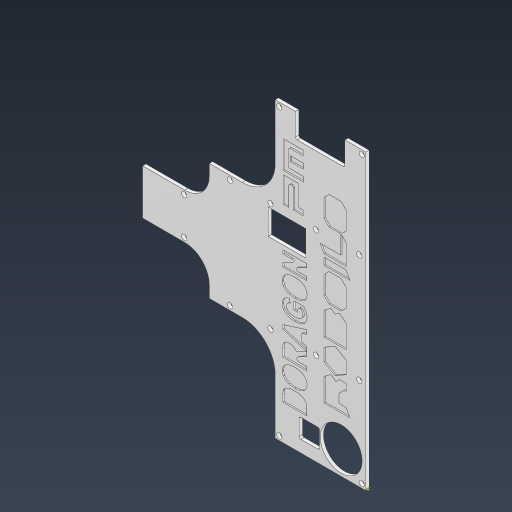
# Autodesk Inventor part: ceil
Saved by Autodesk Inventor 2023 (Build 270158000, 158)
## iProperties
Created: 2024-05-26
Part Number: ceil
Material: ABS Plastic
Document SubType Name: Modeling
Designer: szymo
Density: 1.06 g/cm^3
Appearance: Smooth - White
Mass: 26.6149 g
Surface Area: 293.171 cm^2
Volume: 25.1084 cm^3
TOTAL MASS: 0.0
Author: szymo
Autodesk Inventor part; units mm, degrees
ref_plane "YZ Plane" through (0, 0, 0) normal (1, 0, 0) x (0, 1, 0)
ref_plane "XZ Plane" through (0, 0, 0) normal (0, 1, 0) x (-1, 0, 0)
ref_plane "Work Plane1" through (-50.5, 0, 0) normal (0, 0, 1) x (1, 0, 0)
sketch "Sketch3" plane through (-50.5, 0, 0) normal (0, 0, 1) x (1, 0, 0)
  line L0 (135.5648, 0) -> (135.5648, 5.2284) projected
  line L1 (0, 5) -> (134.493, 5) projected
  line L2 (0, 0) -> (0, 5) projected
  line L3 (0, 71) -> (135.5648, 71) projected
  line L4 (0, 71) -> (0, 66) projected
  line L5 (0, 66) -> (135.5648, 66) projected
  line L6 (135.5648, 71) -> (135.5648, 66) projected
  line L7 (131.5648, 119.5) -> (134.5648, 119.5) projected
  line L8 (135.5648, 124.5) -> (135.5648, 120.5) projected
  line L9 (135.5648, 124.5) -> (51.5, 124.5) projected
  line L10 (86.5, 123.5) -> (129.5648, 123.5) projected
  line L11 (80.5, 122.5) -> (80.5, 120.5) projected
  line L12 (81.5, 119.5) -> (84.5, 119.5) projected
  line L13 (85.5, 122.5) -> (85.5, 120.5) projected
  line L14 (51.5, 123.5) -> (79.5, 123.5) projected
  line L15 (130.5648, 122.5) -> (130.5648, 120.5) projected
  line L16 (120.8148, 112) -> (120.8148, 123) projected
  line L17 (120.8148, 123) -> (94.8148, 123) projected
  line L18 (94.8148, 123) -> (94.8148, 112) projected
  line L19 (94.8148, 112) -> (120.8148, 112) projected
  line L20 (130.5648, -51.5) -> (130.5648, -49.5) projected
  line L21 (51.5, -52.5) -> (79.5, -52.5) projected
  line L22 (85.5, -51.5) -> (85.5, -49.5) projected
  line L23 (131.5648, -48.5) -> (134.5648, -48.5) projected
  line L24 (80.5, -51.5) -> (80.5, -49.5) projected
  line L25 (86.5, -52.5) -> (129.5648, -52.5) projected
  line L26 (135.5648, -53.5) -> (51.5, -53.5) projected
  line L27 (135.5648, -53.5) -> (135.5648, -49.5) projected
  line L28 (81.5, -48.5) -> (84.5, -48.5) projected
  line L29 (95.5648, -45.8) -> (95.5648, -35.2) projected
  line L30 (106.8648, -35.2) -> (95.5648, -35.2) projected
  line L31 (106.8648, -35.2) -> (106.8648, -45.8) projected
  line L32 (95.5648, -45.8) -> (106.8648, -45.8) projected
  circle A0 centre (90.4898, -49.075) radius 1.675 projected
  circle A1 centre (124.5398, -49.075) radius 1.675 projected
  line L33 (126.3648, -33.5) -> (126.3648, -45.5) projected
  line L34 (126.3648, -45.5) -> (114.7648, -45.5) projected
  line L35 (114.7648, -45.5) -> (114.7648, -33.5) projected
  line L36 (114.7648, -33.5) -> (86.8648, -33.5) projected
  line L37 (86.8648, -33.5) -> (86.8648, -52.5) projected
  line L38 (86.8648, -52.5) -> (128.0648, -52.5) projected
  line L39 (128.0648, -52.5) -> (128.0648, -33.5) projected
  line L40 (128.0648, -33.5) -> (126.3648, -33.5) projected
  line L41 (126.3648, -32.7) -> (114.7648, -32.7) projected
  line L42 (114.7648, -32.7) -> (114.7648, -45.5) projected
  line L43 (114.7648, -45.5) -> (126.3648, -45.5) projected
  line L44 (126.3648, -45.5) -> (126.3648, -32.7) projected
  line L45 (80.5, -53.5) -> (135.5648, -53.5)
  line L46 (135.5648, -53.5) -> (135.5648, 124.5)
  line L47 (135.5648, 124.5) -> (80.5, 124.5)
  line L48 (80.5, 124.5) -> (80.5, -53.5)
  line L49 (0, 22) -> (80.5, 22)
  line L50 (80.5, 22) -> (80.5, 49.5)
  line L51 (80.5, 49.5) -> (0, 49.5)
  line L52 (0, 49.5) -> (0, 22)
  line L53 (80.5, 22) -> (50.5, 22)
  line L54 (50.5, 22) -> (50.5, 0)
  line L55 (50.5, 0) -> (80.5, 0)
  line L56 (80.5, 0) -> (80.5, 22)
  line L57 (80.5, 46.5815) -> (80.5, 71)
  line L58 (80.5, 71) -> (50.5, 71)
  line L59 (50.5, 71) -> (50.5, 49.5)
  arc A2 (97.9124, 50.9) -> (98.0124, 51) centre (97.9124, 51) ccw projected
  line L60 (77.4124, 50.9) -> (97.9124, 50.9) projected
  arc A3 (77.3124, 51) -> (77.4124, 50.9) centre (77.4124, 51) ccw projected
  line L61 (77.3124, 65.5) -> (77.3124, 51) projected
  arc A4 (77.4124, 65.6) -> (77.3124, 65.5) centre (77.4124, 65.5) ccw projected
  line L62 (97.9124, 65.6) -> (77.4124, 65.6) projected
  arc A5 (98.0124, 65.5) -> (97.9124, 65.6) centre (97.9124, 65.5) ccw projected
  line L63 (98.0124, 51) -> (98.0124, 65.5) projected
  line L64 (96.2124, 63.7) -> (96.2124, 52.8) projected
  arc A6 (96.2124, 63.7) -> (95.9124, 64) centre (95.9124, 63.7) ccw projected
  line L65 (95.9124, 64) -> (95.8124, 64) projected
  line L66 (95.8124, 64) -> (95.3509, 64.55) projected
  line L67 (95.3509, 64.55) -> (94.9739, 64.55) projected
  line L68 (94.9739, 64.55) -> (94.5124, 64) projected
  line L69 (94.5124, 64) -> (90.8124, 64) projected
  line L70 (90.8124, 64) -> (90.8124, 64.35) projected
  line L71 (90.8124, 64.35) -> (89.5124, 64.35) projected
  line L72 (89.5124, 64) -> (89.5124, 64.35) projected
  line L73 (89.5124, 64) -> (85.8124, 64) projected
  line L74 (85.8124, 64) -> (85.8124, 64.35) projected
  line L75 (85.8124, 64.35) -> (84.5124, 64.35) projected
  line L76 (84.5124, 64) -> (84.5124, 64.35) projected
  line L77 (84.5124, 64) -> (80.8124, 64) projected
  line L78 (80.8124, 64) -> (80.3509, 64.55) projected
  line L79 (80.3509, 64.55) -> (79.9739, 64.55) projected
  line L80 (79.9739, 64.55) -> (79.5124, 64) projected
  line L81 (79.5124, 64) -> (79.4124, 64) projected
  arc A7 (79.4124, 64) -> (79.1124, 63.7) centre (79.4124, 63.7) ccw projected
  line L82 (79.1124, 63.7) -> (79.1124, 52.8) projected
  arc A8 (79.1124, 52.8) -> (79.4124, 52.5) centre (79.4124, 52.8) ccw projected
  line L83 (79.4124, 52.5) -> (79.5124, 52.5) projected
  line L84 (79.5124, 52.5) -> (79.9739, 51.95) projected
  line L85 (80.3509, 51.95) -> (79.9739, 51.95) projected
  line L86 (80.3509, 51.95) -> (80.8124, 52.5) projected
  line L87 (80.8124, 52.5) -> (84.5124, 52.5) projected
  line L88 (84.5124, 52.5) -> (84.5124, 52.15) projected
  line L89 (85.8124, 52.15) -> (84.5124, 52.15) projected
  line L90 (85.8124, 52.5) -> (85.8124, 52.15) projected
  line L91 (85.8124, 52.5) -> (89.5124, 52.5) projected
  line L92 (89.5124, 52.5) -> (89.5124, 52.15) projected
  line L93 (90.8124, 52.15) -> (89.5124, 52.15) projected
  line L94 (90.8124, 52.5) -> (90.8124, 52.15) projected
  line L95 (90.8124, 52.5) -> (94.5124, 52.5) projected
  line L96 (94.5124, 52.5) -> (94.9739, 51.95) projected
  line L97 (95.3509, 51.95) -> (94.9739, 51.95) projected
  line L98 (95.3509, 51.95) -> (95.8124, 52.5) projected
  line L99 (95.8124, 52.5) -> (95.9124, 52.5) projected
  arc A9 (95.9124, 52.5) -> (96.2124, 52.8) centre (95.9124, 52.8) ccw projected
  line L100 (78.1624, 55.35) -> (78.8624, 55.35) projected
  line L101 (78.8624, 55.35) -> (78.8624, 61.15) projected
  line L102 (78.1624, 61.15) -> (78.8624, 61.15) projected
  line L103 (78.1624, 61.15) -> (78.1624, 55.35) projected
  line L104 (97.1624, 61.15) -> (97.1624, 55.35) projected
  line L105 (96.4624, 61.15) -> (97.1624, 61.15) projected
  line L106 (96.4624, 55.35) -> (96.4624, 61.15) projected
  line L107 (96.4624, 55.35) -> (97.1624, 55.35) projected
  arc A10 (76.8124, 51) -> (77.4124, 50.4) centre (77.4124, 51) ccw
  line L108 (77.4124, 50.4) -> (97.9124, 50.4)
  arc A11 (97.9124, 50.4) -> (98.5124, 51) centre (97.9124, 51) ccw
  line L109 (98.5124, 51) -> (98.5124, 65.5)
  arc A12 (98.5124, 65.5) -> (97.9124, 66.1) centre (97.9124, 65.5) ccw
  line L110 (97.9124, 66.1) -> (77.4124, 66.1)
  arc A13 (77.4124, 66.1) -> (76.8124, 65.5) centre (77.4124, 65.5) ccw
  line L111 (76.8124, 65.5) -> (76.8124, 51)
  line L112 (95.0648, -34.7) -> (95.0648, -46.3)
  line L113 (95.0648, -46.3) -> (107.3648, -46.3)
  line L114 (107.3648, -46.3) -> (107.3648, -34.7)
  line L115 (107.3648, -34.7) -> (95.0648, -34.7)
  line L116 (114.2648, -45.5) -> (114.2648, -32.2)
  line L117 (114.2648, -32.2) -> (126.8648, -32.2)
  line L118 (126.8648, -32.2) -> (126.8648, -45.5)
  line L119 (126.3648, -46) -> (114.7648, -46)
  line L120 (92.8148, 110) -> (92.8148, 125)
  line L121 (92.8148, 125) -> (122.8148, 125)
  line L122 (122.8148, 125) -> (122.8148, 110)
  line L123 (122.8148, 110) -> (92.8148, 110)
  line L124 (114.2648, -45.5) -> (114.2648, -46)
  line L125 (114.2648, -46) -> (114.7648, -46)
  line L126 (126.3648, -46) -> (126.8648, -46)
  line L127 (126.8648, -46) -> (126.8648, -45.5)
  line L128 (51.5, -53.5) -> (51.5, -52.5) projected
  line L129 (51.5, 124.5) -> (51.5, 123.5) projected
  circle A14 centre (105.3205, 68.5) radius 1.75 projected
  circle A15 centre (53, 68.5) radius 1.75 projected
  circle A16 centre (77.648, 2.5) radius 1.75 projected
  circle A17 centre (131.5519, 2.5) radius 1.75 projected
  line L130 (50.5, 27) -> (0, 27) projected
  line L131 (0, 27) -> (0, 22) projected
  line L132 (50.5, 22) -> (0, 22) projected
  line L133 (50.5, 27) -> (50.5, 22) projected
  line L134 (50.5, 44.5) -> (0, 44.5) projected
  line L135 (50.5, 44.5) -> (50.5, 49.5) projected
  line L136 (50.5, 49.5) -> (0, 49.5) projected
  line L137 (0, 44.5) -> (0, 49.5) projected
  line L138 (50.5, 0) -> (40.5, 0)
  line L139 (40.5, 0) -> (40.5, 22)
  line L140 (40.5, 22) -> (50.5, 22)
  line L141 (50.5, 22) -> (50.5, 0)
  line L142 (50.5, 49.5) -> (40.5, 49.5)
  line L143 (40.5, 49.5) -> (40.5, 71)
  line L144 (40.5, 71) -> (50.5, 71)
  line L145 (50.5, 71) -> (50.5, 49.5)
  ellipse E0 centre (134.493, 7) end of major axis (136.8024, 7) minor radius 2 (134.493, 5) -> (135.5648, 5.2284) ccw projected
  circle A18 centre (25.25, 47) radius 1.75 projected
  circle A19 centre (25.25, 24.5) radius 1.75 projected
  line L146 (0, 0) -> (3.5, 0) projected
  line L147 (3.5, 0) -> (47, 0) projected
  line L148 (47, 0) -> (135.5648, 0) projected
  circle A20 centre (105.3205, 2.5) radius 1.75 projected
  circle A21 centre (53, 2.5) radius 1.75 projected
  arc A22 (81.5, -48.5) -> (80.5, -49.5) centre (81.5, -49.5) ccw projected
  arc A23 (79.5, -52.5) -> (80.5, -51.5) centre (79.5, -51.5) ccw projected
  arc A24 (135.5648, -49.5) -> (134.5648, -48.5) centre (134.5648, -49.5) ccw projected
  arc A25 (131.5648, -48.5) -> (130.5648, -49.5) centre (131.5648, -49.5) ccw projected
  arc A26 (129.5648, -52.5) -> (130.5648, -51.5) centre (129.5648, -51.5) ccw projected
  arc A27 (85.5, -51.5) -> (86.5, -52.5) centre (86.5, -51.5) ccw projected
  arc A28 (85.5, -49.5) -> (84.5, -48.5) centre (84.5, -49.5) ccw projected
  circle A29 centre (133.0648, -51) radius 1.75 projected
  circle A30 centre (83, -51) radius 1.75 projected
  arc A31 (86.5, 123.5) -> (85.5, 122.5) centre (86.5, 122.5) ccw projected
  arc A32 (130.5648, 122.5) -> (129.5648, 123.5) centre (129.5648, 122.5) ccw projected
  arc A33 (134.5648, 119.5) -> (135.5648, 120.5) centre (134.5648, 120.5) ccw projected
  arc A34 (80.5, 120.5) -> (81.5, 119.5) centre (81.5, 120.5) ccw projected
  arc A35 (84.5, 119.5) -> (85.5, 120.5) centre (84.5, 120.5) ccw projected
  arc A36 (130.5648, 120.5) -> (131.5648, 119.5) centre (131.5648, 120.5) ccw projected
  arc A37 (80.5, 122.5) -> (79.5, 123.5) centre (79.5, 122.5) ccw projected
  circle A38 centre (133.0648, 122) radius 1.75 projected
  circle A39 centre (83, 122) radius 1.75 projected
  point P0 (122.8148, 124.5)
  point P1 (92.8148, 124.5)
  point P2 (0, 44)
  point P3 (50.5, 44)
  point P4 (122.8148, 124.5)
  point P5 (122.8148, 123.5)
  point P6 (92.8148, 123.5)
  point P7 (92.8148, 124.5)
  point P8 (80.5, 123.5)
  point P9 (50.5, 66)
  point P10 (50.5, 5)
  point P11 (80.5, -52.5)
  point P12 (80.5, 66)
  point P13 (80.5, 5)
  point P14 (135.5648, 5)
  point P15 (80.5, 22)
  point P16 (50.5, 27)
  point P17 (0, 27)
  point P18 (80.5, -51.5)
  point P19 (77.0807, 66)
  point P20 (80.5, 66.1)
  point P21 (135.5648, 5.2284)
  point P22 (80.5, 50.4)
  point P23 (40.5, 5)
  point P24 (135.5648, 119.5)
  point P25 (80.5, 119.5)
  dimension "d16" = 0.5
  dimension "d17" = 0.5
  dimension "d18" = 0.5
  dimension "d19" = 0.5
  dimension "d20" = 2
  dimension "d191" = 10
  dimension "d192" = 10
  constraints: 86 end point, 12 parallel, 8 point on circle, 7 perpendicular, 7 point on line, 6 horizontal, 4 centre point, 2 collinear, 2 vertical, 17 other
  measures "d16" distance between parallel lines of L61 L111
  measures "d17" distance between parallel lines of L29 L112
  measures "d18" distance between parallel lines of L42 L116
  measures "d19" distance between parallel lines of L34 L119
  measures "d20" distance between parallel lines of L18 L120
  measures "d191" distance between parallel lines of L139 L54
  measures "d192" distance between parallel lines of L59 L143
extrude "Extrusion2" add sketch "Sketch3" along normal blind 2 contours L148 L48 L1 E0 L0 | L46 A24 L23 A25 L20 A26 L25 L39 L40 L118 L117 L116 L36 L37 A27 L22 A28 L28 A22 L48 L148 | E0 L1 L48 L108 A11 L109 A12 L5 L46 | L27 L26 L48 L24 A22 L28 A28 L22 A27 L25 A26 L20 A25 L23 A24 | L55 L54 L1 L48 | L5 A12 L110 L48 L3 L6 | L1 L54 L49 L48 | L138 L139 L1 L54 | A12 L109 A11 L108 L48 L60 A2 L63 A5 L62 L5 | L5 L48 L110 A12 | L3 L48 A34 L12 A35 L13 A31 L10 L120 L123 L122 A32 L15 A36 L7 A33 L46 | L1 L139 L49 L54 | L49 L133 L130 L52 L134 L135 L51 L48 | L48 L62 A4 L61 A3 L60 L108 A10 L111 A13 L5 | L5 A13 L110 L48 | L48 L110 A13 L5 L59 L3 | A33 L7 A36 L15 A32 L10 L122 L9 L8 | L49 L52 L130 L133 | A13 L111 A10 L108 L48 L51 L59 L5 | L62 A5 L63 A2 L60 L48 L86 L87 L88 L89 L90 L91 L92 L93 L94 L95 L96 L97 L98 L99 A9 L64 A6 L65 L66 L67 L68 L69 L70 L71 L72 L73 L74 L75 L76 L77 L78 | L48 L78 L79 L80 L81 A7 L82 A8 L83 L84 L85 L86 L60 A3 L61 A4 L62 | L59 L5 L143 L3 | L11 L48 L9 L120 L10 A31 L13 A35 L12 A34 | L59 L51 L143 L5 | L78 L77 L76 L75 L74 L73 L72 L71 L70 L69 L68 L67 L66 L65 A6 L64 A9 L99 L98 L97 L96 L95 L94 L93 L92 L91 L90 L89 L88 L87 L86 L48 | L48 L86 L85 L84 L83 A8 L82 A7 L81 L80 L79 L78 | L135 L134 L52 L51 | L25 L37 L36 L116 L124 L125 L119 L126 L127 L118 L40 L39 | A0 | A1 | L103 L102 L101 L100 | L104 L107 L106 L105 | A14 | A15 | A16 | A17 | A18 | A19 | A20 | A21 | A29 | A30 | A38 | A39
fillet "Fillet2" radius 1 10 edges at (44.5648, -46.3, 1) (44.5648, -34.7, 1) (56.8648, -34.7, 1) (56.8648, -46.3, 1) (63.7648, -46, 1) (63.7648, -32.2, 1) (76.3648, -32.2, 1) (76.3648, -46, 1) (42.3148, 110, 1) (72.3148, 110, 1)
fillet "Fillet3" radius 20 2 edges at (30, 71, 1) (30, 0, 1)
sketch "Sketch4" plane through (-50.5, 0, 2) normal (0, 0, 1) x (1, 0, 0)
  line L0 (130.5648, -51.5) -> (130.5648, -49.5) projected
  line L1 (51.5, -52.5) -> (79.5, -52.5) projected
  line L2 (85.5, -51.5) -> (85.5, -49.5) projected
  line L3 (131.5648, -48.5) -> (134.5648, -48.5) projected
  line L4 (80.5, -51.5) -> (80.5, -49.5) projected
  line L5 (86.5, -52.5) -> (129.5648, -52.5) projected
  line L6 (135.5648, -53.5) -> (51.5, -53.5) projected
  line L7 (135.5648, -53.5) -> (135.5648, -49.5) projected
  line L8 (81.5, -48.5) -> (84.5, -48.5) projected
  line L9 (131.5648, 119.5) -> (134.5648, 119.5) projected
  line L10 (135.5648, 124.5) -> (135.5648, 120.5) projected
  line L11 (135.5648, 124.5) -> (51.5, 124.5) projected
  line L12 (86.5, 123.5) -> (129.5648, 123.5) projected
  line L13 (80.5, 122.5) -> (80.5, 120.5) projected
  line L14 (81.5, 119.5) -> (84.5, 119.5) projected
  line L15 (85.5, 122.5) -> (85.5, 120.5) projected
  line L16 (51.5, 123.5) -> (79.5, 123.5) projected
  line L17 (130.5648, 122.5) -> (130.5648, 120.5) projected
  line L18 (51.5, 124.5) -> (51.5, 123.5) projected
  line L19 (51.5, -53.5) -> (51.5, -52.5) projected
  line L20 (50.5, 27) -> (0, 27) projected
  line L21 (0, 27) -> (0, 22) projected
  line L22 (50.5, 22) -> (0, 22) projected
  line L23 (50.5, 27) -> (50.5, 22) projected
  line L24 (50.5, 44.5) -> (0, 44.5) projected
  line L25 (50.5, 44.5) -> (50.5, 49.5) projected
  line L26 (50.5, 49.5) -> (0, 49.5) projected
  line L27 (0, 44.5) -> (0, 49.5) projected
  circle A0 centre (77.648, 68.5) radius 1.75 projected
  circle A1 centre (105.3205, 68.5) radius 1.75 projected
  circle A2 centre (53, 68.5) radius 1.75 projected
  circle A3 centre (131.5519, 68.5) radius 1.75 projected
  line L28 (0, 71) -> (0, 66) projected
  line L29 (0, 66) -> (134.493, 66) projected
  line L30 (135.5648, 71) -> (135.5648, 65.7716) projected
  circle A4 centre (77.648, 2.5) radius 1.75 projected
  circle A5 centre (105.3205, 2.5) radius 1.75 projected
  circle A6 centre (53, 2.5) radius 1.75 projected
  circle A7 centre (131.5519, 2.5) radius 1.75 projected
  line L31 (135.5648, 0) -> (135.5648, 5.2284) projected
  line L32 (0, 5) -> (134.493, 5) projected
  line L33 (0, 0) -> (0, 5) projected
  ellipse E0 centre (134.493, 64) end of major axis (136.8024, 64) minor radius 2 (135.5648, 65.7716) -> (134.493, 66) ccw projected
  ellipse E1 centre (134.493, 7) end of major axis (136.8024, 7) minor radius 2 (134.493, 5) -> (135.5648, 5.2284) ccw projected
  circle A8 centre (25.25, 47) radius 1.75 projected
  circle A9 centre (25.25, 24.5) radius 1.75 projected
  line L34 (0, 71) -> (3.5, 71) projected
  line L35 (47, 71) -> (135.5648, 71) projected
  line L36 (3.5, 71) -> (47, 71) projected
  line L37 (0, 0) -> (3.5, 0) projected
  line L38 (3.5, 0) -> (47, 0) projected
  line L39 (47, 0) -> (135.5648, 0) projected
  arc A10 (86.5, 123.5) -> (85.5, 122.5) centre (86.5, 122.5) ccw projected
  arc A11 (130.5648, 122.5) -> (129.5648, 123.5) centre (129.5648, 122.5) ccw projected
  arc A12 (134.5648, 119.5) -> (135.5648, 120.5) centre (134.5648, 120.5) ccw projected
  arc A13 (81.5, -48.5) -> (80.5, -49.5) centre (81.5, -49.5) ccw projected
  arc A14 (79.5, -52.5) -> (80.5, -51.5) centre (79.5, -51.5) ccw projected
  arc A15 (135.5648, -49.5) -> (134.5648, -48.5) centre (134.5648, -49.5) ccw projected
  arc A16 (131.5648, -48.5) -> (130.5648, -49.5) centre (131.5648, -49.5) ccw projected
  arc A17 (129.5648, -52.5) -> (130.5648, -51.5) centre (129.5648, -51.5) ccw projected
  arc A18 (85.5, -51.5) -> (86.5, -52.5) centre (86.5, -51.5) ccw projected
  arc A19 (85.5, -49.5) -> (84.5, -48.5) centre (84.5, -49.5) ccw projected
  circle A20 centre (133.0648, -51) radius 1.75 projected
  circle A21 centre (83, -51) radius 1.75 projected
  arc A22 (80.5, 120.5) -> (81.5, 119.5) centre (81.5, 120.5) ccw projected
  arc A23 (84.5, 119.5) -> (85.5, 120.5) centre (84.5, 120.5) ccw projected
  arc A24 (130.5648, 120.5) -> (131.5648, 119.5) centre (131.5648, 120.5) ccw projected
  arc A25 (80.5, 122.5) -> (79.5, 123.5) centre (79.5, 122.5) ccw projected
  circle A26 centre (133.0648, 122) radius 1.75 projected
  circle A27 centre (83, 122) radius 1.75 projected
  point P0 (50.5, 0)
  point P1 (83, -51)
  point P2 (133.0648, -51)
  point P3 (0, 44)
  point P4 (50.5, 44)
  point P5 (50.5, 27)
  point P6 (0, 27)
  constraints: 10 coincident, 2 other
hole "Hole2" at (32.5, -51, 2) at (82.5648, -51, 2) at (82.5648, 122, 2) at (32.5, 122, 2) at (54.8205, 68.5, 2) at (2.5, 2.5, 2) at (2.5, 68.5, 2) at (54.8205, 2.5, 2) at (81.0519, 2.5, 2) at (81.0519, 68.5, 2) at (27.148, 68.5, 2) at (27.148, 2.5, 2) at (-25.25, 24.5, 2) at (-25.25, 47, 2) direction (0, 0, -1) diameter 3.2 end through all clearance for "Countersunk Flat Head Screw ISO 2009/7046" size "M2.5" standard "ISO"
fillet "Fillet4" radius 15 2 edges at (-10, 22, 1) (-10, 49.5, 1)
sketch "Sketch8" plane through (-50.5, 0, 2) normal (0, 0, 1) x (1, 0, 0)
  line L0 (74.2124, 66) -> (82.148, 66) projected
  arc A0 (76.2124, 64) -> (74.2124, 66) centre (74.2124, 64) ccw projected
  line L1 (76.2124, 50.5) -> (76.2124, 64) projected
  line L2 (99.1124, 50.5) -> (76.2124, 50.5) projected
  line L3 (99.1124, 66) -> (99.1124, 50.5) projected
  line L4 (97.3737, 66) -> (99.1124, 66) projected
  line L5 (97.3737, 66) -> (82.148, 66) projected
  line L6 (97.7124, 65.2) -> (77.6124, 65.2) projected
  line L7 (97.7124, 51.9) -> (97.7124, 65.2) projected
  line L8 (77.6124, 51.9) -> (97.7124, 51.9) projected
  line L9 (77.6124, 65.2) -> (77.6124, 51.9) projected
  line L10 (76.2124, 64) -> (76.2124, 66)
  point P0 (50.5, 0)
  constraints: 2 end point, 1 perpendicular, 1 point on circle, 1 point on line, 1 tangent
extrude "Extrusion6" cut sketch "Sketch8" against normal blind 10 contours L0 L5 L4 L3 L2 L1 L10 | L7 L8 L9 L6
sketch "Sketch5" plane through (-50.5, 0, 2) normal (0, 0, 1) x (1, 0, 0)
  line L0 (80.5, -53.5) -> (135.5648, -53.5) projected
  line L1 (135.5648, -53.5) -> (135.5648, 124.5) projected
  line L2 (60.5, 71) -> (40.5, 71) projected
  line L3 (25.5, 49.5) -> (0, 49.5) projected
  line L4 (0, 49.5) -> (0, 22) projected
  line L5 (0, 22) -> (25.5, 22) projected
  line L6 (105.3205, -33.9758) -> (105.3205, 49.8239) construction
  line L7 (105.3205, 49.8239) -> (79.4085, 49.8239) construction
  line L8 (79.4085, 49.8239) -> (79.4085, -33.9758) construction
  line L9 (79.4085, -33.9758) -> (105.3205, -33.9758) construction
  line L10 (110.1651, 28.6458) -> (110.1651, 14.5717) projected
  line L11 (119.2148, -10.52) -> (122.2141, -7.4431) projected
  line L12 (122.2141, -7.4431) -> (123.5648, -7.4431) projected
  line L13 (123.5648, -7.4431) -> (123.5648, -3.1151) projected
  line L14 (123.5648, -3.1151) -> (119.5551, -3.1151) projected
  line L15 (119.5551, -3.1151) -> (117.3584, -5.3021) projected
  line L16 (117.3584, -5.3021) -> (114.3535, -3.0659) projected
  line L17 (114.3535, -3.0659) -> (110.1651, -6.1782) projected
  line L18 (110.1651, -6.1782) -> (110.1651, -20.0711) projected
  line L19 (110.1651, -20.0711) -> (125.9602, -20.0711) projected
  line L20 (125.9602, -20.0711) -> (123.4807, -15.7431) projected
  line L21 (123.4807, -15.7431) -> (119.2148, -15.7431) projected
  line L22 (119.2148, -15.7431) -> (119.2148, -10.52) projected
  line L23 (114.6271, -7.6036) -> (115.8612, -8.5098) projected
  line L24 (115.8612, -8.5098) -> (115.8612, -15.7431) projected
  line L25 (115.8612, -15.7431) -> (113.4584, -15.7431) projected
  line L26 (113.4584, -15.7431) -> (113.4584, -8.4973) projected
  line L27 (113.4584, -8.4973) -> (114.6271, -7.6036) projected
  line L28 (123.5648, 1.4254) -> (123.5648, 9.1617) projected
  line L29 (123.5648, 9.1617) -> (116.8649, 13.0299) projected
  line L30 (116.8649, 13.0299) -> (110.1651, 9.1617) projected
  line L31 (110.1651, 9.1617) -> (110.1651, 1.4254) projected
  line L32 (110.1651, 1.4254) -> (116.8649, -2.4427) projected
  line L33 (116.8649, -2.4427) -> (123.5648, 1.4254) projected
  circle A0 centre (116.8649, 5.2936) radius 3.3 projected
  line L34 (123.5848, 14.5717) -> (123.5848, 28.6458) projected
  line L35 (123.5848, 28.6458) -> (119.3867, 31.747) projected
  line L36 (119.3867, 31.747) -> (116.875, 29.8983) projected
  line L37 (116.875, 29.8983) -> (114.3632, 31.747) projected
  line L38 (114.3632, 31.747) -> (110.1651, 28.6458) projected
  line L39 (110.1651, 28.6458) -> (110.1651, 14.5717) projected
  line L40 (110.1651, 14.5717) -> (123.5848, 14.5717) projected
  line L41 (115.3489, 26.1486) -> (115.3489, 18.8997) projected
  line L42 (115.3489, 18.8997) -> (113.4785, 18.8997) projected
  line L43 (113.4785, 18.8997) -> (113.4785, 26.1539) projected
  line L44 (113.4785, 26.1539) -> (114.3691, 26.9374) projected
  line L45 (114.3691, 26.9374) -> (115.3489, 26.1486) projected
  line L46 (118.4011, 18.8997) -> (118.4011, 26.1486) projected
  line L47 (118.4011, 26.1486) -> (119.3808, 26.9374) projected
  line L48 (119.3808, 26.9374) -> (120.2715, 26.1539) projected
  line L49 (120.2715, 26.1539) -> (120.2715, 18.8997) projected
  line L50 (120.2715, 18.8997) -> (118.4011, 18.8997) projected
  line L51 (120.494, 33.3579) -> (123.5648, 36.4286) projected
  line L52 (123.5648, 36.4286) -> (123.5648, 47.4441) projected
  line L53 (123.5648, 47.4441) -> (120.494, 50.5148) projected
  line L54 (120.494, 50.5148) -> (113.2358, 50.5148) projected
  line L55 (113.2358, 50.5148) -> (110.1651, 47.4441) projected
  line L56 (110.1651, 47.4441) -> (110.1651, 36.4286) projected
  line L57 (110.1651, 36.4286) -> (113.2358, 33.3579) projected
  line L58 (113.2358, 33.3579) -> (120.494, 33.3579) projected
  line L59 (120.2715, 37.686) -> (113.4584, 37.686) projected
  line L60 (113.4584, 37.686) -> (113.4584, 46.1868) projected
  line L61 (113.4584, 46.1868) -> (120.2715, 46.1868) projected
  line L62 (120.2715, 46.1868) -> (120.2715, 37.686) projected
  line L63 (125.9586, 52.2145) -> (123.5013, 56.5425) projected
  line L64 (123.5013, 56.5425) -> (110.1651, 56.5425) projected
  line L65 (110.1651, 56.5425) -> (110.1651, 52.2145) projected
  line L66 (110.1651, 52.2145) -> (125.9586, 52.2145) projected
  line L67 (123.5648, 88.0003) -> (120.494, 91.071) projected
  line L68 (120.494, 91.071) -> (113.2358, 91.071) projected
  line L69 (113.2358, 91.071) -> (110.1651, 88.0003) projected
  line L70 (110.1651, 88.0003) -> (110.1651, 76.9848) projected
  line L71 (110.1651, 76.9848) -> (113.2358, 73.9141) projected
  line L72 (113.2358, 73.9141) -> (120.2715, 73.9141) projected
  line L73 (120.2715, 73.9141) -> (120.2715, 62.7008) projected
  line L74 (120.2715, 62.7008) -> (107.738, 62.7008) projected
  line L75 (107.738, 62.7008) -> (110.2396, 58.3727) projected
  line L76 (110.2396, 58.3727) -> (123.5848, 58.3727) projected
  line L77 (123.5848, 58.3727) -> (123.5848, 70.8415) projected
  line L78 (123.5848, 70.8415) -> (120.5032, 73.9232) projected
  line L79 (120.5032, 73.9232) -> (123.5648, 76.9848) projected
  line L80 (123.5648, 76.9848) -> (123.5648, 88.0003) projected
  line L81 (120.2715, 78.2421) -> (113.4584, 78.2421) projected
  line L82 (113.4584, 78.2421) -> (113.4584, 86.743) projected
  line L83 (113.4584, 86.743) -> (120.2715, 86.743) projected
  line L84 (120.2715, 86.743) -> (120.2715, 78.2421) projected
  line L85 (91.5024, 71.975) -> (97.5262, 71.975) projected
  line L86 (97.5262, 71.975) -> (97.5262, 74.9242) projected
  line L87 (97.5262, 74.9242) -> (94.45, 74.9242) projected
  line L88 (94.45, 74.9242) -> (94.45, 87.525) projected
  line L89 (94.45, 87.525) -> (85.5, 87.525) projected
  line L90 (85.5, 87.525) -> (85.5, 71.975) projected
  line L91 (85.5, 71.975) -> (88.675, 71.975) projected
  line L92 (88.675, 71.975) -> (88.675, 84.4887) projected
  line L93 (88.675, 84.4887) -> (91.5024, 84.4887) projected
  line L94 (91.5024, 84.4887) -> (91.5024, 71.975) projected
  line L95 (85.5, 106.5) -> (85.5, 89.825) projected
  line L96 (85.5, 89.825) -> (97.6, 89.825) projected
  line L97 (97.6, 89.825) -> (97.6, 92.775) projected
  line L98 (97.6, 92.775) -> (88.6, 92.775) projected
  line L99 (88.6, 92.775) -> (88.6, 103.4705) projected
  line L100 (88.6, 103.4705) -> (97.5254, 103.4705) projected
  line L101 (97.5254, 103.4705) -> (97.5254, 106.5) projected
  line L102 (97.5254, 106.5) -> (85.5, 106.5) projected
  line L103 (89.7, 99.675) -> (89.7, 96.575) projected
  line L104 (89.7, 96.575) -> (97.6, 96.575) projected
  line L105 (97.6, 96.575) -> (97.6, 99.675) projected
  line L106 (97.6, 99.675) -> (89.7, 99.675) projected
  line L107 (80.5, -20) -> (80.5, -53.5) projected
  line L108 (80.5, 124.5) -> (80.5, 91) projected
  arc A1 (60.5, 71) -> (80.5, 91) centre (60.5, 91) ccw projected
  circle A2 centre (105.3205, 2.5) radius 1.6 projected
  line L109 (40.5, 71) -> (40.5, 64.5) projected
  line L110 (40.5, 7) -> (40.5, 0) projected
  arc A3 (25.5, 49.5) -> (40.5, 64.5) centre (25.5, 64.5) ccw projected
  arc A4 (40.5, 7) -> (25.5, 22) centre (25.5, 7) ccw projected
  line L111 (40.5, 0) -> (60.5, 0) projected
  arc A5 (80.5, -20) -> (60.5, 0) centre (60.5, -20) ccw projected
  line L112 (135.5648, 124.5) -> (122.8148, 124.5) projected
  line L113 (122.8148, 124.5) -> (122.8148, 111) projected
  arc A6 (121.8148, 110) -> (122.8148, 111) centre (121.8148, 111) ccw projected
  line L114 (121.8148, 110) -> (93.8148, 110) projected
  arc A7 (92.8148, 111) -> (93.8148, 110) centre (93.8148, 111) ccw projected
  line L115 (92.8148, 111) -> (92.8148, 124.5) projected
  line L116 (92.8148, 124.5) -> (80.5, 124.5) projected
  line L117 (85.1145, -32.172) -> (85.1145, -28.0055)
  spline S0 degree 2 poles (85.1145, -28.0055) (85.1145, -26.5908) (85.3908, -25.8504) knots 0 0 0 1 1 1
  spline S1 degree 2 poles (85.3908, -25.8504) (85.7666, -24.8557) (87.6896, -23.4411) (90.4636, -22.7006) (92.5082, -22.7006) knots 0 0 0 1 2 3 3 3
  spline S2 degree 2 poles (92.5082, -22.7006) (94.2986, -22.7006) (95.5916, -23.0432) knots 0 0 0 1 1 1
  spline S3 degree 2 poles (95.5916, -23.0432) (97.172, -23.4742) (98.1557, -24.2589) knots 0 0 0 1 1 1
  spline S4 degree 2 poles (98.1557, -24.2589) (98.8961, -24.8557) (99.305, -25.8614) knots 0 0 0 1 1 1
  spline S5 degree 2 poles (99.305, -25.8614) (99.6145, -26.6129) (99.6145, -27.8839) knots 0 0 0 1 1 1
  line L118 (99.6145, -27.8839) -> (99.6145, -32.172)
  line L119 (99.6145, -32.172) -> (85.1145, -32.172)
  line L120 (87.568, -29.8843) -> (97.161, -29.8843)
  line L121 (97.161, -29.8843) -> (97.161, -28.1823)
  spline S6 degree 2 poles (97.161, -28.1823) (97.161, -27.2318) (97.0173, -26.8008) knots 0 0 0 1 1 1
  spline S7 degree 2 poles (97.0173, -26.8008) (96.8405, -26.2482) (96.0005, -25.5188) (94.0444, -25.0546) (92.3645, -25.0546) knots 0 0 0 1 2 3 3 3
  spline S8 degree 2 poles (92.3645, -25.0546) (90.6846, -25.0546) (88.8942, -25.5188) (87.8885, -26.3477) (87.7117, -26.9887) knots 0 0 0 1 2 3 3 3
  spline S9 degree 2 poles (87.7117, -26.9887) (87.568, -27.4639) (87.568, -28.8565) knots 0 0 0 1 1 1
  line L122 (87.568, -28.8565) -> (87.568, -29.8843)
  spline S10 degree 2 poles (92.4529, -21.2307) (90.2425, -21.2307) (88.7395, -20.7113) knots 0 0 0 1 1 1
  spline S11 degree 2 poles (88.7395, -20.7113) (87.6343, -20.3245) (85.866, -18.9872) (85.4461, -18.2025) knots 0 0 0 1 2 2 2
  spline S12 degree 2 poles (85.4461, -18.2025) (84.8714, -17.1415) (84.8714, -15.76) knots 0 0 0 1 1 1
  spline S13 degree 2 poles (84.8714, -15.76) (84.8714, -13.2623) (88.85, -10.2562) (92.3866, -10.2562) knots 0 0 0 1 2 2 2
  spline S14 degree 2 poles (92.3866, -10.2562) (95.89, -10.2562) (99.8576, -13.2402) (99.8576, -15.7269) knots 0 0 0 1 2 2 2
  spline S15 degree 2 poles (99.8576, -15.7269) (99.8576, -18.2467) (95.9121, -21.2307) (92.4529, -21.2307) knots 0 0 0 1 2 2 2
  spline S16 degree 2 poles (92.3534, -18.8767) (94.818, -18.8767) (97.3599, -17.0973) (97.3599, -15.7269) knots 0 0 0 1 2 2 2
  spline S17 degree 2 poles (97.3599, -15.7269) (97.3599, -14.3675) (94.8401, -12.6103) (92.3203, -12.6103) knots 0 0 0 1 2 2 2
  spline S18 degree 2 poles (92.3203, -12.6103) (89.8226, -12.6103) (87.3691, -14.3233) (87.3691, -15.7269) knots 0 0 0 1 2 2 2
  spline S19 degree 2 poles (87.3691, -15.7269) (87.3691, -17.1415) (89.8557, -18.8767) (92.3534, -18.8767) knots 0 0 0 1 2 2 2
  line L123 (99.6145, -8.4769) -> (85.1145, -8.4769)
  line L124 (85.1145, -8.4769) -> (85.1145, -3.6693)
  spline S20 degree 2 poles (85.1145, -3.6693) (85.1145, -1.8568) (85.8992, -0.2101) (87.8885, 0.7735) (89.1816, 0.7735) knots 0 0 0 1 2 3 3 3
  spline S21 degree 2 poles (89.1816, 0.7735) (90.8062, 0.7735) (92.9392, -0.7185) (93.2155, -2.2105) knots 0 0 0 1 2 2 2
  spline S22 degree 2 poles (93.2155, -2.2105) (93.7681, -1.47) (95.0943, -0.5085) (96.7852, 0.3093) knots 0 0 0 1 2 2 2
  line L125 (96.7852, 0.3093) -> (99.6145, 1.6908)
  line L126 (99.6145, 1.6908) -> (99.6145, -1.039)
  line L127 (99.6145, -1.039) -> (96.4537, -2.6857)
  spline S23 degree 2 poles (96.4537, -2.6857) (94.7627, -3.5699) (93.8896, -4.2109) (93.5581, -4.9403) (93.5581, -5.725) knots 0 0 0 1 2 3 3 3
  line L128 (93.5581, -5.725) -> (93.5581, -6.1892)
  line L129 (93.5581, -6.1892) -> (99.6145, -6.1892)
  line L130 (99.6145, -6.1892) -> (99.6145, -8.4769)
  line L131 (91.2483, -6.1892) -> (91.2483, -4.4982)
  spline S24 degree 2 poles (91.2483, -4.4982) (91.2483, -2.8626) (90.8946, -2.0447) (90.0215, -1.5806) (89.3695, -1.5806) knots 0 0 0 1 2 3 3 3
  spline S25 degree 2 poles (89.3695, -1.5806) (88.64, -1.5806) (87.7338, -2.1884) (87.6122, -2.741) knots 0 0 0 1 2 2 2
  spline S26 degree 2 poles (87.6122, -2.741) (87.568, -3.0173) (87.568, -4.4098) knots 0 0 0 1 1 1
  line L132 (87.568, -4.4098) -> (87.568, -6.1892)
  line L133 (87.568, -6.1892) -> (91.2483, -6.1892)
  line L134 (99.6145, 13.1294) -> (99.6145, 10.6428)
  line L135 (99.6145, 10.6428) -> (96.3211, 9.6592)
  line L136 (96.3211, 9.6592) -> (96.3211, 5.139)
  line L137 (96.3211, 5.139) -> (99.6145, 4.1996)
  line L138 (99.6145, 4.1996) -> (99.6145, 1.7792)
  line L139 (99.6145, 1.7792) -> (85.1145, 6.1778)
  line L140 (85.1145, 6.1778) -> (85.1145, 8.6092)
  line L141 (85.1145, 8.6092) -> (99.6145, 13.1294)
  line L142 (93.8675, 8.9297) -> (88.4964, 7.3714)
  line L143 (88.4964, 7.3714) -> (93.8675, 5.8352)
  line L144 (93.8675, 5.8352) -> (93.8675, 8.9297)
  line L145 (94.2986, 19.5948) -> (91.8451, 19.5948)
  line L146 (91.8451, 19.5948) -> (91.8451, 24.5128)
  line L147 (91.8451, 24.5128) -> (97.6141, 24.5128)
  spline S27 degree 2 poles (97.6141, 24.5128) (98.5093, 23.7944) (99.8576, 21.0757) (99.8576, 19.6721) knots 0 0 0 1 2 2 2
  spline S28 degree 2 poles (99.8576, 19.6721) (99.8576, 17.9038) (97.9457, 15.2624) (94.398, 13.9362) (92.3203, 13.9362) knots 0 0 0 1 2 3 3 3
  spline S29 degree 2 poles (92.3203, 13.9362) (90.0547, 13.9362) (86.5291, 15.4172) (85.5897, 16.8428) knots 0 0 0 1 2 2 2
  spline S30 degree 2 poles (85.5897, 16.8428) (84.8714, 17.937) (84.8714, 19.5505) knots 0 0 0 1 1 1
  spline S31 degree 2 poles (84.8714, 19.5505) (84.8714, 21.6614) (87.137, 24.0265) (89.1374, 24.3691) knots 0 0 0 1 2 2 2
  line L148 (89.1374, 24.3691) -> (89.6789, 22.1035)
  spline S32 degree 2 poles (89.6789, 22.1035) (88.6069, 21.8604) (87.3691, 20.5452) (87.3691, 19.5505) knots 0 0 0 1 2 2 2
  spline S33 degree 2 poles (87.3691, 19.5505) (87.3691, 18.0585) (89.8005, 16.2903) (92.1987, 16.2903) knots 0 0 0 1 2 2 2
  spline S34 degree 2 poles (92.1987, 16.2903) (94.7738, 16.2903) (97.3599, 18.0807) (97.3599, 19.5284) knots 0 0 0 1 2 2 2
  spline S35 degree 2 poles (97.3599, 19.5284) (97.3599, 20.2468) (96.6416, 21.6835) (96.1332, 22.203) knots 0 0 0 1 2 2 2
  line L149 (96.1332, 22.203) -> (94.2986, 22.203)
  line L150 (94.2986, 22.203) -> (94.2986, 19.5948)
  spline S36 degree 2 poles (92.4529, 26.1595) (90.2425, 26.1595) (88.7395, 26.679) knots 0 0 0 1 1 1
  spline S37 degree 2 poles (88.7395, 26.679) (87.6343, 27.0658) (85.866, 28.4031) (85.4461, 29.1877) knots 0 0 0 1 2 2 2
  spline S38 degree 2 poles (85.4461, 29.1877) (84.8714, 30.2487) (84.8714, 31.6302) knots 0 0 0 1 1 1
  spline S39 degree 2 poles (84.8714, 31.6302) (84.8714, 34.1279) (88.85, 37.134) (92.3866, 37.134) knots 0 0 0 1 2 2 2
  spline S40 degree 2 poles (92.3866, 37.134) (95.89, 37.134) (99.8576, 34.15) (99.8576, 31.6634) knots 0 0 0 1 2 2 2
  spline S41 degree 2 poles (99.8576, 31.6634) (99.8576, 29.1435) (95.9121, 26.1595) (92.4529, 26.1595) knots 0 0 0 1 2 2 2
  spline S42 degree 2 poles (92.3534, 28.5136) (94.818, 28.5136) (97.3599, 30.2929) (97.3599, 31.6634) knots 0 0 0 1 2 2 2
  spline S43 degree 2 poles (97.3599, 31.6634) (97.3599, 33.0227) (94.8401, 34.78) (92.3203, 34.78) knots 0 0 0 1 2 2 2
  spline S44 degree 2 poles (92.3203, 34.78) (89.8226, 34.78) (87.3691, 33.0669) (87.3691, 31.6634) knots 0 0 0 1 2 2 2
  spline S45 degree 2 poles (87.3691, 31.6634) (87.3691, 30.2487) (89.8557, 28.5136) (92.3534, 28.5136) knots 0 0 0 1 2 2 2
  line L151 (99.6145, 38.9355) -> (85.1145, 38.9355)
  line L152 (85.1145, 38.9355) -> (85.1145, 41.1458)
  line L153 (85.1145, 41.1458) -> (94.8401, 45.7986)
  line L154 (94.8401, 45.7986) -> (85.1145, 45.7986)
  line L155 (85.1145, 45.7986) -> (85.1145, 47.9095)
  line L156 (85.1145, 47.9095) -> (99.6145, 47.9095)
  line L157 (99.6145, 47.9095) -> (99.6145, 45.6329)
  line L158 (99.6145, 45.6329) -> (90.1099, 41.0464)
  line L159 (90.1099, 41.0464) -> (99.6145, 41.0464)
  line L160 (99.6145, 41.0464) -> (99.6145, 38.9355)
  point P0 (50.5, 0)
  point P1 (79.4085, -20)
  constraints: 2 point on line, 2 other
extrude "Extrusion4" cut sketch "Sketch5" against normal blind 0.8 contours L38 L37 L36 L35 L34 L40 L10 | L22 L21 L20 L19 L18 L17 L16 L15 L14 L13 L12 L11 | L33 L32 L31 L30 L29 L28 | L58 L57 L56 L55 L54 L53 L52 L51 | L66 L65 L64 L63 | L80 L79 L78 L77 L76 L75 L74 L73 L72 L71 L70 L69 L68 L67 | L94 L93 L92 L91 L90 L89 L88 L87 L86 L85 | L102 L101 L100 L99 L98 L97 L96 L95 | L106 L105 L104 L103 | L117 S0 S1 S2 S3 S4 S5 L118 L119 | S10 S11 S12 S13 S14 S15 | L123 L124 S20 S21 S22 L125 L126 L127 S23 L128 L129 L130 | L134 L135 L136 L137 L138 L139 L140 L141 | L145 L146 L147 S27 S28 S29 S30 S31 L148 S32 S33 S34 S35 L149 L150 | S36 S37 S38 S39 S40 S41 | L151 L152 L153 L154 L155 L156 L157 L158 L159 L160
sketch "Sketch9" plane through (-50.5, 0, 2) normal (0, 0, 1) x (1, 0, 0)
  line L0 (60.5, 71) -> (40.5, 71) projected
  line L1 (40.5, 71) -> (40.5, 64.5) projected
  arc A0 (25.5, 49.5) -> (40.5, 64.5) centre (25.5, 64.5) ccw projected
  line L2 (25.5, 49.5) -> (0, 49.5) projected
  line L3 (0, 49.5) -> (0, 22) projected
  line L4 (0, 22) -> (25.5, 22) projected
  arc A1 (40.5, 7) -> (25.5, 22) centre (25.5, 7) ccw projected
  line L5 (40.5, 7) -> (40.5, 0) projected
  line L6 (40.5, 0) -> (60.5, 0) projected
  arc A2 (80.5, -20) -> (60.5, 0) centre (60.5, -20) ccw projected
  line L7 (80.5, -20) -> (80.5, -53.5) projected
  line L8 (80.5, -53.5) -> (135.5648, -53.5) projected
  line L9 (135.5648, -53.5) -> (135.5648, 124.5) projected
  line L10 (135.5648, 124.5) -> (122.8148, 124.5) projected
  line L11 (122.8148, 124.5) -> (122.8148, 111) projected
  arc A3 (121.8148, 110) -> (122.8148, 111) centre (121.8148, 111) ccw projected
  line L12 (121.8148, 110) -> (93.8148, 110) projected
  arc A4 (92.8148, 111) -> (93.8148, 110) centre (93.8148, 111) ccw projected
  line L13 (92.8148, 111) -> (92.8148, 124.5) projected
  line L14 (92.8148, 124.5) -> (80.5, 124.5) projected
  line L15 (80.5, 124.5) -> (80.5, 91) projected
  arc A5 (60.5, 71) -> (80.5, 91) centre (60.5, 91) ccw projected
  line L16 (114.2648, -45) -> (114.2648, -33.2) projected
  arc A6 (115.2648, -32.2) -> (114.2648, -33.2) centre (115.2648, -33.2) ccw projected
  line L17 (115.2648, -32.2) -> (125.8648, -32.2) projected
  arc A7 (126.8648, -33.2) -> (125.8648, -32.2) centre (125.8648, -33.2) ccw projected
  line L18 (126.8648, -33.2) -> (126.8648, -45) projected
  arc A8 (125.8648, -46) -> (126.8648, -45) centre (125.8648, -45) ccw projected
  line L19 (125.8648, -46) -> (115.2648, -46) projected
  arc A9 (114.2648, -45) -> (115.2648, -46) centre (115.2648, -45) ccw projected
  line L20 (96.0648, -34.7) -> (106.3648, -34.7) projected
  arc A10 (107.3648, -35.7) -> (106.3648, -34.7) centre (106.3648, -35.7) ccw projected
  line L21 (107.3648, -35.7) -> (107.3648, -45.3) projected
  arc A11 (106.3648, -46.3) -> (107.3648, -45.3) centre (106.3648, -45.3) ccw projected
  line L22 (106.3648, -46.3) -> (96.0648, -46.3) projected
  arc A12 (95.0648, -45.3) -> (96.0648, -46.3) centre (96.0648, -45.3) ccw projected
  line L23 (95.0648, -45.3) -> (95.0648, -35.7) projected
  arc A13 (96.0648, -34.7) -> (95.0648, -35.7) centre (96.0648, -35.7) ccw projected
  circle A14 centre (25.25, 47) radius 1.6 projected
  circle A15 centre (77.648, 2.5) radius 1.6 projected
  circle A16 centre (131.5519, 68.5) radius 1.6 projected
  circle A17 centre (105.3205, 2.5) radius 1.6 projected
  circle A18 centre (53, 2.5) radius 1.6 projected
  circle A19 centre (83, 122) radius 1.6 projected
  circle A20 centre (133.0648, -51) radius 1.6 projected
  circle A21 centre (83, -51) radius 1.6 projected
  circle A22 centre (133.0648, 122) radius 1.6 projected
  circle A23 centre (105.3205, 68.5) radius 1.6 projected
  circle A24 centre (53, 68.5) radius 1.6 projected
  circle A25 centre (131.5519, 2.5) radius 1.6 projected
  circle A26 centre (77.648, 68.5) radius 1.6 projected
  circle A27 centre (25.25, 24.5) radius 1.6 projected
  line L24 (99.1124, 66) -> (99.1124, 50.5) projected
  line L25 (99.1124, 50.5) -> (76.2124, 50.5) projected
  line L26 (76.2124, 50.5) -> (76.2124, 66) projected
  line L27 (76.2124, 66) -> (99.1124, 66) projected
  line L28 (99.6145, 41.0464) -> (99.6145, 38.9355) projected
  line L29 (99.6145, 38.9355) -> (85.1145, 38.9355) projected
  line L30 (85.1145, 38.9355) -> (85.1145, 41.1458) projected
  line L31 (85.1145, 41.1458) -> (94.8401, 45.7986) projected
  line L32 (94.8401, 45.7986) -> (85.1145, 45.7986) projected
  line L33 (85.1145, 45.7986) -> (85.1145, 47.9095) projected
  line L34 (85.1145, 47.9095) -> (99.6145, 47.9095) projected
  line L35 (99.6145, 47.9095) -> (99.6145, 45.6329) projected
  line L36 (99.6145, 45.6329) -> (90.1099, 41.0464) projected
  line L37 (90.1099, 41.0464) -> (99.6145, 41.0464) projected
  line L38 (123.5648, -3.1151) -> (123.5648, -7.4431) projected
  line L39 (123.5648, -7.4431) -> (122.2141, -7.4431) projected
  line L40 (122.2141, -7.4431) -> (119.2148, -10.52) projected
  line L41 (119.2148, -10.52) -> (119.2148, -15.7431) projected
  line L42 (119.2148, -15.7431) -> (123.4807, -15.7431) projected
  line L43 (123.4807, -15.7431) -> (125.9602, -20.0711) projected
  line L44 (125.9602, -20.0711) -> (110.1651, -20.0711) projected
  line L45 (110.1651, -20.0711) -> (110.1651, -6.1782) projected
  line L46 (110.1651, -6.1782) -> (114.3535, -3.0659) projected
  line L47 (114.3535, -3.0659) -> (117.3584, -5.3021) projected
  line L48 (117.3584, -5.3021) -> (119.5551, -3.1151) projected
  line L49 (119.5551, -3.1151) -> (123.5648, -3.1151) projected
  line L50 (110.1651, 52.2145) -> (110.1651, 56.5425) projected
  line L51 (110.1651, 56.5425) -> (123.5013, 56.5425) projected
  line L52 (123.5013, 56.5425) -> (125.9586, 52.2145) projected
  line L53 (125.9586, 52.2145) -> (110.1651, 52.2145) projected
  line L54 (97.6, 99.675) -> (97.6, 96.575) projected
  line L55 (97.6, 96.575) -> (89.7, 96.575) projected
  line L56 (89.7, 96.575) -> (89.7, 99.675) projected
  line L57 (89.7, 99.675) -> (97.6, 99.675) projected
  line L58 (110.1651, 88.0003) -> (113.2358, 91.071) projected
  line L59 (113.2358, 91.071) -> (120.494, 91.071) projected
  line L60 (120.494, 91.071) -> (123.5648, 88.0003) projected
  line L61 (123.5648, 88.0003) -> (123.5648, 76.9848) projected
  line L62 (123.5648, 76.9848) -> (120.5032, 73.9232) projected
  line L63 (120.5032, 73.9232) -> (123.5848, 70.8415) projected
  line L64 (123.5848, 70.8415) -> (123.5848, 58.3727) projected
  line L65 (123.5848, 58.3727) -> (110.2396, 58.3727) projected
  line L66 (110.2396, 58.3727) -> (107.738, 62.7008) projected
  line L67 (107.738, 62.7008) -> (120.2715, 62.7008) projected
  line L68 (120.2715, 62.7008) -> (120.2715, 73.9141) projected
  line L69 (120.2715, 73.9141) -> (113.2358, 73.9141) projected
  line L70 (113.2358, 73.9141) -> (110.1651, 76.9848) projected
  line L71 (110.1651, 76.9848) -> (110.1651, 88.0003) projected
  line L72 (110.1651, 9.1617) -> (116.8649, 13.0299) projected
  line L73 (116.8649, 13.0299) -> (123.5648, 9.1617) projected
  line L74 (123.5648, 9.1617) -> (123.5648, 1.4254) projected
  line L75 (123.5648, 1.4254) -> (116.8649, -2.4427) projected
  line L76 (116.8649, -2.4427) -> (110.1651, 1.4254) projected
  line L77 (110.1651, 1.4254) -> (110.1651, 9.1617) projected
  line L78 (120.494, 50.5148) -> (123.5648, 47.4441) projected
  line L79 (123.5648, 47.4441) -> (123.5648, 36.4286) projected
  line L80 (123.5648, 36.4286) -> (120.494, 33.3579) projected
  line L81 (120.494, 33.3579) -> (113.2358, 33.3579) projected
  line L82 (113.2358, 33.3579) -> (110.1651, 36.4286) projected
  line L83 (110.1651, 36.4286) -> (110.1651, 47.4441) projected
  line L84 (110.1651, 47.4441) -> (113.2358, 50.5148) projected
  line L85 (113.2358, 50.5148) -> (120.494, 50.5148) projected
  line L86 (97.6, 92.775) -> (97.6, 89.825) projected
  line L87 (97.6, 89.825) -> (85.5, 89.825) projected
  line L88 (85.5, 89.825) -> (85.5, 106.5) projected
  line L89 (85.5, 106.5) -> (97.5254, 106.5) projected
  line L90 (97.5254, 106.5) -> (97.5254, 103.4705) projected
  line L91 (97.5254, 103.4705) -> (88.6, 103.4705) projected
  line L92 (88.6, 103.4705) -> (88.6, 92.775) projected
  line L93 (88.6, 92.775) -> (97.6, 92.775) projected
  line L94 (94.45, 74.9242) -> (97.5262, 74.9242) projected
  line L95 (97.5262, 74.9242) -> (97.5262, 71.975) projected
  line L96 (97.5262, 71.975) -> (91.5024, 71.975) projected
  line L97 (91.5024, 71.975) -> (91.5024, 84.4887) projected
  line L98 (91.5024, 84.4887) -> (88.675, 84.4887) projected
  line L99 (88.675, 84.4887) -> (88.675, 71.975) projected
  line L100 (88.675, 71.975) -> (85.5, 71.975) projected
  line L101 (85.5, 71.975) -> (85.5, 87.525) projected
  line L102 (85.5, 87.525) -> (94.45, 87.525) projected
  line L103 (94.45, 87.525) -> (94.45, 74.9242) projected
  line L104 (123.5848, 14.5717) -> (110.1651, 14.5717) projected
  line L105 (110.1651, 14.5717) -> (110.1651, 28.6458) projected
  line L106 (110.1651, 28.6458) -> (114.3632, 31.747) projected
  line L107 (114.3632, 31.747) -> (116.875, 29.8983) projected
  line L108 (116.875, 29.8983) -> (119.3867, 31.747) projected
  line L109 (119.3867, 31.747) -> (123.5848, 28.6458) projected
  line L110 (123.5848, 28.6458) -> (123.5848, 14.5717) projected
  line L111 (99.6145, -32.172) -> (85.1145, -32.172) projected
  line L112 (85.1145, -32.172) -> (85.1145, -28.0055) projected
  line L113 (99.6145, -27.8839) -> (99.6145, -32.172) projected
  line L114 (99.6145, -6.1892) -> (99.6145, -8.4769) projected
  line L115 (99.6145, -8.4769) -> (85.1145, -8.4769) projected
  line L116 (85.1145, -8.4769) -> (85.1145, -3.6693) projected
  line L117 (96.7852, 0.3093) -> (99.6145, 1.6908) projected
  line L118 (99.6145, 1.6908) -> (99.6145, -1.039) projected
  line L119 (99.6145, -1.039) -> (96.4537, -2.6857) projected
  line L120 (93.5581, -5.725) -> (93.5581, -6.1892) projected
  line L121 (93.5581, -6.1892) -> (99.6145, -6.1892) projected
  line L122 (85.1145, 8.6092) -> (99.6145, 13.1294) projected
  line L123 (99.6145, 13.1294) -> (99.6145, 10.6428) projected
  line L124 (99.6145, 10.6428) -> (96.3211, 9.6592) projected
  line L125 (96.3211, 9.6592) -> (96.3211, 5.139) projected
  line L126 (96.3211, 5.139) -> (99.6145, 4.1996) projected
  line L127 (99.6145, 4.1996) -> (99.6145, 1.7792) projected
  line L128 (99.6145, 1.7792) -> (85.1145, 6.1778) projected
  line L129 (85.1145, 6.1778) -> (85.1145, 8.6092) projected
  line L130 (94.2986, 22.203) -> (94.2986, 19.5948) projected
  line L131 (94.2986, 19.5948) -> (91.8451, 19.5948) projected
  line L132 (91.8451, 19.5948) -> (91.8451, 24.5128) projected
  line L133 (91.8451, 24.5128) -> (97.6141, 24.5128) projected
  line L134 (89.1374, 24.3691) -> (89.6789, 22.1035) projected
  line L135 (96.1332, 22.203) -> (94.2986, 22.203) projected
  line L136 (115.2648, -45) -> (125.8648, -33.2) construction
  line L137 (125.8648, -45) -> (115.2648, -33.2) construction
  circle A28 centre (120.5648, -39.1) radius 12.7
  point P0 (50.5, 0)
  dimension "d195" = 0.5
  constraints: 4 end point, 1 centre point, 1 coincident, 1 midpoint, 31 other
  measures "d195" distance edge to line of A28 L21
extrude "Extrusion7" cut sketch "Sketch9" against normal blind 10 contours A28
sketch "Sketch10" plane through (-50.5, 0, 2) normal (0, 0, 1) x (1, 0, 0)
  line L0 (97.161, -29.8843) -> (97.161, -28.1823) projected
  spline S0 degree 2 poles (97.161, -28.1823) (97.161, -27.2318) (97.0173, -26.8008) knots 0 0 0 1 1 1 projected
  spline S1 degree 2 poles (97.0173, -26.8008) (96.8405, -26.2482) (96.0005, -25.5188) (94.0444, -25.0546) (92.3645, -25.0546) knots 0 0 0 0.333333 0.666667 1 1 1 projected
  spline S2 degree 2 poles (92.3645, -25.0546) (90.6846, -25.0546) (88.8942, -25.5188) (87.8885, -26.3477) (87.7117, -26.9887) knots 0 0 0 0.333333 0.666667 1 1 1 projected
  spline S3 degree 2 poles (87.7117, -26.9887) (87.568, -27.4639) (87.568, -28.8565) knots 0 0 0 1 1 1 projected
  line L1 (87.568, -28.8565) -> (87.568, -29.8843) projected
  line L2 (87.568, -29.8843) -> (97.161, -29.8843) projected
  spline S4 degree 2 poles (97.3599, -15.7269) (97.3599, -14.3675) (94.8401, -12.6103) (92.3203, -12.6103) knots 0 0 0 0.5 1 1 1 projected
  spline S5 degree 2 poles (92.3203, -12.6103) (89.8226, -12.6103) (87.3691, -14.3233) (87.3691, -15.7269) knots 0 0 0 0.5 1 1 1 projected
  spline S6 degree 2 poles (87.3691, -15.7269) (87.3691, -17.1415) (89.8557, -18.8767) (92.3534, -18.8767) knots 0 0 0 0.5 1 1 1 projected
  spline S7 degree 2 poles (92.3534, -18.8767) (94.818, -18.8767) (97.3599, -17.0973) (97.3599, -15.7269) knots 0 0 0 0.5 1 1 1 projected
  spline S8 degree 2 poles (91.2483, -4.4982) (91.2483, -2.8626) (90.8946, -2.0447) (90.0215, -1.5806) (89.3695, -1.5806) knots 0 0 0 0.333333 0.666667 1 1 1 projected
  spline S9 degree 2 poles (89.3695, -1.5806) (88.64, -1.5806) (87.7338, -2.1884) (87.6122, -2.741) knots 0 0 0 0.5 1 1 1 projected
  spline S10 degree 2 poles (87.6122, -2.741) (87.568, -3.0173) (87.568, -4.4098) knots 0 0 0 1 1 1 projected
  line L3 (87.568, -4.4098) -> (87.568, -6.1892) projected
  line L4 (87.568, -6.1892) -> (91.2483, -6.1892) projected
  line L5 (91.2483, -6.1892) -> (91.2483, -4.4982) projected
  line L6 (88.4964, 7.3714) -> (93.8675, 5.8352) projected
  line L7 (93.8675, 5.8352) -> (93.8675, 8.9297) projected
  line L8 (93.8675, 8.9297) -> (88.4964, 7.3714) projected
  spline S11 degree 2 poles (97.3599, 31.6634) (97.3599, 33.0227) (94.8401, 34.78) (92.3203, 34.78) knots 0 0 0 0.5 1 1 1 projected
  spline S12 degree 2 poles (92.3203, 34.78) (89.8226, 34.78) (87.3691, 33.0669) (87.3691, 31.6634) knots 0 0 0 0.5 1 1 1 projected
  spline S13 degree 2 poles (87.3691, 31.6634) (87.3691, 30.2487) (89.8557, 28.5136) (92.3534, 28.5136) knots 0 0 0 0.5 1 1 1 projected
  spline S14 degree 2 poles (92.3534, 28.5136) (94.818, 28.5136) (97.3599, 30.2929) (97.3599, 31.6634) knots 0 0 0 0.5 1 1 1 projected
  line L9 (113.4584, 86.743) -> (113.4584, 78.2421) projected
  line L10 (113.4584, 78.2421) -> (120.2715, 78.2421) projected
  line L11 (120.2715, 78.2421) -> (120.2715, 86.743) projected
  line L12 (120.2715, 86.743) -> (113.4584, 86.743) projected
  line L13 (113.4584, 46.1868) -> (113.4584, 37.686) projected
  line L14 (113.4584, 37.686) -> (120.2715, 37.686) projected
  line L15 (120.2715, 37.686) -> (120.2715, 46.1868) projected
  line L16 (120.2715, 46.1868) -> (113.4584, 46.1868) projected
  line L17 (113.4785, 18.8997) -> (115.3489, 18.8997) projected
  line L18 (115.3489, 18.8997) -> (115.3489, 26.1486) projected
  line L19 (115.3489, 26.1486) -> (114.3691, 26.9374) projected
  line L20 (114.3691, 26.9374) -> (113.4785, 26.1539) projected
  line L21 (113.4785, 26.1539) -> (113.4785, 18.8997) projected
  line L22 (119.3808, 26.9374) -> (118.4011, 26.1486) projected
  line L23 (118.4011, 26.1486) -> (118.4011, 18.8997) projected
  line L24 (118.4011, 18.8997) -> (120.2715, 18.8997) projected
  line L25 (120.2715, 18.8997) -> (120.2715, 26.1539) projected
  line L26 (120.2715, 26.1539) -> (119.3808, 26.9374) projected
  circle A0 centre (116.8649, 5.2936) radius 3.3 projected
  line L27 (115.8612, -15.7431) -> (115.8612, -8.5098) projected
  line L28 (115.8612, -8.5098) -> (114.6271, -7.6036) projected
  line L29 (114.6271, -7.6036) -> (113.4584, -8.4973) projected
  line L30 (113.4584, -8.4973) -> (113.4584, -15.7431) projected
  line L31 (113.4584, -15.7431) -> (115.8612, -15.7431) projected
  point P0 (50.5, 0)
  constraints: 15 other
extrude "Extrusion8" cut sketch "Sketch10" against normal up to surface (0.8 mm away)
fillet "Fillet5" radius 1 15 edges at (41.0024, 84.4887, 1.6) (38.175, 84.4887, 1.6) (43.95, 74.9242, 1.6) (38.1, 92.775, 1.6) (38.1, 103.4705, 1.6) (70.0032, 73.9232, 1.6) (69.7715, 73.9141, 1.6) (39.6099, 41.0464, 1.6) (44.3401, 45.7986, 1.6) (43.0581, -6.1892, 1.6) (42.7155, -2.2105, 1.6) (45.8211, 5.139, 1.6) (45.8211, 9.6592, 1.6) (43.7986, 22.203, 1.6) (45.6332, 22.203, 1.6)
body "Solid2"
